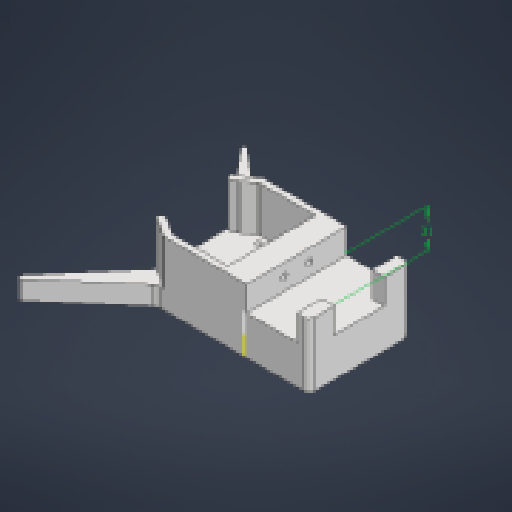
# Autodesk Inventor part: KeChan
Saved by Autodesk Inventor 2027 (Build 310192060, 192F)
## iProperties
Created: 2026-08-23
Part Number: KeChan
Material: Generic
Document SubType Name: Modeling
Designer: trtrn
Density: 1 g/cm^3
Appearance: Default
Author: trtrn
Autodesk Inventor part; units mm, degrees
ref_plane "YZ Plane" through (0, 0, 0) normal (1, 0, 0) x (0, 1, 0)
ref_plane "XZ Plane" through (0, 0, 0) normal (0, 1, 0) x (-1, 0, 0)
ref_plane "XY Plane" through (0, 0, 0) normal (0, 0, 1) x (1, 0, 0)
sketch "Sketch38" plane through (0, 0, 0) normal (0, 1, 0) x (-1, 0, 0)
  line L0 (40, 40) -> (-40, 40)
  line L1 (-40, 40) -> (-40, -40)
  line L2 (-40, -40) -> (40, -40)
  line L3 (40, -40) -> (40, 40)
  line L4 (40, 40) -> (-40, -40) construction
  line L5 (-40, 40) -> (40, -40) construction
  point P0 (0, 0)
  dimension "d203" = 80
  dimension "d204" = 80
  constraints: 12 end point, 2 midpoint, 2 parallel, 1 horizontal, 1 perpendicular
  measures "d203" distance of L2.end L1.end
  measures "d204" distance of L1.end L0.end
extrude "Extrusion36" add sketch "Sketch38" along normal blind 15
sketch "Sketch39" plane through (0, 0, 0) normal (0, -1, 0) x (1, 0, 0)
  line L0 (-35, -35) -> (35, -35)
  line L1 (35, -35) -> (35, 35)
  line L2 (35, 35) -> (-35, 35)
  line L3 (-35, 35) -> (-35, -35)
  line L4 (-35, -35) -> (35, 35) construction
  line L5 (35, -35) -> (-35, 35) construction
  point P0 (0, 0)
  dimension "d207" = 70
  dimension "d208" = 70
  constraints: 12 end point, 2 midpoint, 2 parallel, 1 horizontal, 1 perpendicular
  measures "d207" distance of L2.end L1.end
  measures "d208" distance of L1.end L0.end
extrude "Extrusion37" cut sketch "Sketch39" against normal blind 6
fillet "Fillet5" radius 8 4 edges at (-40, 7.5, -40) (40, 7.5, -40) (40, 7.5, 40) (-40, 7.5, 40)
sketch "Sketch43" plane through (0, 15, 0) normal (0, 1, 0) x (1, 0, 0)
  arc A0 (-32, 40) -> (-40, 32) centre (-32, 32) ccw projected
  arc A1 (-26.7833, 38.0652) -> (-38.0652, 26.7833) centre (-32, 32) ccw
  line L0 (-38.0652, 26.7833) -> (-90.0848, 87.2644)
  line L1 (-87.2644, 90.0848) -> (-26.7833, 38.0652)
  line L2 (0, 0) -> (-32, 32) construction
  arc A2 (-87.2644, 90.0848) -> (-90.0848, 87.2644) centre (-88.5685, 88.5685) ccw
  line L3 (32, 40) -> (-32, 40) projected
  line L4 (-29.0329, 40) -> (-32, 40) construction
  line L5 (-40, 32) -> (-40, -32) projected
  point P0 (-107.4247, 107.4247)
  point P1 (-40, 29.0329)
  dimension "d231" = 2
  dimension "d232" = 80
  constraints: 8 end point, 4 point on circle, 4 point on line, 4 tangent, 2 centre point, 1 coincident, 1 collinear, 1 concentric
  measures "d231" radius of A2
  measures "d232" distance of A2.centre A0.centre
extrude "Extrusion40" add sketch "Sketch43" against normal up to surface (15 mm away) contours A0 L5 L0 A2 L1 L3
pattern_circular "Circular Pattern1" count 2 over 90 about axis through (0, -10, 0) along (0, 1, 0) of "Extrusion40"
fillet "Fillet7" radius 8 4 edges at (-29.0329, 7.5, 40) (-40, 7.5, 29.0329) (-40, 7.5, -29.0329) (-29.0329, 7.5, -40)
sketch "Sketch44" plane through (0, 6, 0) normal (0, -1, 0) x (1, 0, 0)
  circle A0 centre (-17.5, 29) radius 1.65
  circle A1 centre (12.5, 29) radius 1.65
  circle A2 centre (12.5, -29) radius 1.65
  circle A3 centre (-17.5, -29) radius 1.65
  point P0 (0, 0)
  constraints: 4 centre point, 4 coincident, 8 other
hole "Hole3" at (-17.5, 6, -29) at (-17.5, 6, 29) at (12.5, 6, 29) at (12.5, 6, -29) direction (0, 1, 0) diameter 4.3 end through all counterbore diameter 7.52 counterbore depth 4
sketch "Sketch46" plane through (40, 0, 32) normal (1, 0, 0) x (0, 0, -1)
  line L0 (64, 15) -> (64, 0) projected
  line L1 (0, 15) -> (64, 15) projected
  line L2 (0, 0) -> (64, 0) projected
  line L3 (0, 0) -> (0, 15) projected
  line L4 (72, 0) -> (72, 15) projected
  line L5 (72, 0) -> (64, 0) projected
  line L6 (64, 15) -> (72, 15) projected
  line L7 (-8, 15) -> (-8, 0) projected
  line L8 (0, 0) -> (-8, 0) projected
  line L9 (-8, 15) -> (0, 15) projected
  line L10 (-8, 15) -> (72, 15)
  line L11 (72, 15) -> (72, 31)
  line L12 (72, 31) -> (-8, 31)
  line L13 (-8, 31) -> (-8, 15)
  point P0 (32, 0)
  dimension "d254" = 31
  constraints: 8 end point, 2 parallel, 1 collinear, 1 horizontal, 1 perpendicular
  measures "d254" distance between parallel lines of L2 L12
extrude "Extrusion41" add sketch "Sketch46" against normal blind 10 contours L6 L4 L5 L0 | L3 L8 L7 L9
sketch "Sketch47" plane through (0, 15, 0) normal (0, 1, 0) x (1, 0, 0)
  line L0 (22, 8) -> (22, 28)
  line L1 (22, -28) -> (22, -8)
  line L2 (-7.5, -35) -> (-2.5, -35)
  line L3 (-2.5, 35) -> (-7.5, 35)
  line L4 (-7.5, -35) -> (22, -35)
  line L5 (22, -35) -> (22, 35)
  line L6 (22, 35) -> (-7.5, 35)
  line L7 (-7.5, -35) -> (-23, -35)
  line L8 (-7.5, 35) -> (-23, 35)
  line L9 (-26.0657, -40) -> (40, -40) projected
  line L10 (40, 40) -> (-26.0657, 40) projected
  arc A0 (-31.2824, 41.9348) -> (-26.0657, 40) centre (-26.0657, 48) ccw projected
  line L11 (-31.2824, 41.9348) -> (-87.2644, 90.0848) projected
  arc A1 (-26.0657, -40) -> (-31.2824, -41.9348) centre (-26.0657, -48) ccw projected
  line L12 (-87.2644, -90.0848) -> (-31.2824, -41.9348) projected
  line L13 (-90.0848, 87.2644) -> (-41.9348, 31.2824) construction
  line L14 (-32.4052, 28.1827) -> (-36.8295, 26.1921)
  arc A2 (-22.6108, 32.1002) -> (-23, 31.3085) centre (-22, 31.3085) ccw construction
  line L15 (-23, 35) -> (-32.4052, 28.1827)
  line L16 (-38.8811, 30.7518) -> (-34.9244, 32.532)
  line L17 (-34.9244, 32.532) -> (-24.6215, 40)
  line L18 (-24.6215, 40) -> (-7.5, 40)
  line L19 (-7.5, 40) -> (27, 40)
  line L20 (27, 40) -> (27, -40)
  line L21 (27, -40) -> (-7.5, -40)
  line L22 (71.2863, 0) -> (-71.2863, 0) construction
  line L23 (-7.5, -35) -> (-23, -35)
  line L24 (-32.4052, -28.1827) -> (-36.8295, -26.1921)
  line L25 (-23, -35) -> (-32.4052, -28.1827)
  line L26 (-38.8811, -30.7518) -> (-34.9244, -32.532)
  line L27 (-34.9244, -32.532) -> (-24.6215, -40)
  line L28 (-36.8295, 26.1921) -> (-40, 24.7656)
  line L29 (-40, 26.0657) -> (-40, -26.0657) projected
  arc A3 (-40, 26.0657) -> (-41.9348, 31.2824) centre (-48, 26.0657) ccw projected
  line L30 (-38.8811, 30.7518) -> (-40.9388, 29.826)
  line L31 (-36.8295, -26.1921) -> (-40, -24.7656)
  line L32 (-38.8811, -30.7518) -> (-40.9388, -29.826)
  arc A4 (-41.9348, -31.2824) -> (-40, -26.0657) centre (-48, -26.0657) ccw projected
  line L33 (-41.9348, -31.2824) -> (-90.0848, -87.2644) construction
  point P0 (0, 0)
  point P1 (22, -8)
  point P2 (27, -40)
  dimension "d248" = 5
  constraints: 54 end point, 8 symmetric about line, 5 collinear, 5 horizontal, 3 point on circle, 2 parallel, 2 perpendicular, 2 vertical, 2 vertical alignment, 1 centre point, 1 midpoint, 1 point on line, 20 other
  measures "d248" distance between parallel lines of L15 L17
extrude "Extrusion42" add sketch "Sketch47" along normal blind 36 contours L0 L5 L6 L3 L8 L15 L14 L28 L29 A3 L30 L16 L17 L10 L20 L9 L27 L26 L32 A4 L31 L24 L25 L7 L2 L4 L1
fillet "Fillet8" radius 2 10 edges at (-40.9388, 33, -29.826) (-40, 33, -24.7656) (-40, 33, 24.7656) (-40.9388, 33, 29.826) (-24.6215, 33, -40) (-34.9244, 33, -32.532) (-32.4052, 33, -28.1827) (-23, 33, -35) (-23, 33, 35) (-24.6215, 33, 40)
fillet "Fillet9" radius 2 2 edges at (-34.9244, 33, 32.532) (-32.4052, 33, 28.1827)
extrude "Extrusion43" add sketch "Sketch46" against normal up to surface (13 mm away) contours L1 L9 L13 L12 L11 L6
extrude "Extrusion44" add sketch "Sketch46" along normal blind 52
sketch "Sketch48" plane through (27, 51, 40) normal (1, 0, 0) x (0, 0, -1)
  line L0 (0, 0) -> (80, 0) projected
  line L1 (80, -20) -> (80, 0) projected
  line L2 (80, -20) -> (0, -20) projected
  line L3 (0, -20) -> (0, 0) projected
  point P0 (40, -51)
extrude "Extrusion45" add sketch "Sketch48" along normal blind 15
sketch "Sketch49" plane through (22, 15, -35) normal (-1, 0, 0) x (0, 0, 1)
  line L0 (35, -15) -> (35, 64.5533) construction
  line L1 (8.9343, -15) -> (61.0657, -15) projected
  point P0 (25, 26)
  point P1 (45, 26)
  point P2 (35, -15)
  dimension "d261" = 20
  dimension "d262" = 41
  constraints: 2 end point, 1 midpoint, 1 symmetric about line, 1 vertical
  measures "d261" distance of point (25, 26) point (45, 26)
  measures "d262" vertical distance of point (35, -15) point (45, 26)
hole "Hole4" at (22, 41, -10) at (22, 41, 10) direction (1, 0, 0) diameter 5.3 end through all counterbore diameter 9 counterbore depth 5
sketch "Sketch50" plane through (92, 31, 40) normal (0, 1, 0) x (1, 0, 0)
  line L0 (-50, 0) -> (0, 0) projected
  line L1 (-50, 80) -> (0, 80) projected
  line L2 (0, 0) -> (-10, 0)
  line L3 (-10, 0) -> (-10, 80)
  line L4 (-10, 80) -> (0, 80)
  line L5 (0, 80) -> (0, 0)
  point P0 (-92, 40)
  dimension "d270" = 10
  constraints: 8 end point, 2 parallel, 1 horizontal, 1 perpendicular, 1 point on line
  measures "d270" distance of L3.end L4.end
extrude "Extrusion46" add sketch "Sketch50" along normal blind 20
fillet "Fillet11" radius 4 2 edges at (92, 25.5, 40) (92, 25.5, -40)
sketch "Sketch51" plane through (0, 0, 0) normal (0, -1, 0) x (1, 0, 0)
  line L0 (30, -35) -> (-35, -35) projected
  line L1 (-35, 35) -> (30, 35) projected
  line L2 (30, -35) -> (87, -35)
  line L3 (87, -35) -> (87, 35)
  line L4 (87, 35) -> (30, 35)
  line L5 (30, 35) -> (30, -35)
  line L6 (92, 36) -> (92, -36) projected
  line L7 (22, -35) -> (22, 35) projected
  line L8 (-159.4505, 0) -> (159.4505, 0) construction
  line L9 (-25, 15) -> (77, 15)
  line L10 (77, 15) -> (77, -15)
  line L11 (77, -15) -> (-25, -15)
  line L12 (-25, -15) -> (-25, 15)
  line L13 (-35, -35) -> (-35, 35) projected
  line L14 (82, 20) -> (-30, 20)
  line L15 (-30, 20) -> (-30, -20)
  line L16 (-30, -20) -> (82, -20)
  line L17 (82, -20) -> (82, 20)
  point P0 (0, 0)
  point P1 (30, -15)
  point P2 (30, -20)
  point P3 (30, 20)
  point P4 (30, 15)
  dimension "d274" = 5
  dimension "d277" = 30
  dimension "d278" = 10
  dimension "d279" = 10
  dimension "d280" = 5
  constraints: 26 end point, 6 parallel, 3 horizontal, 3 perpendicular, 1 collinear, 1 midpoint, 4 other
  measures "d274" distance between parallel lines of L3 L6
  measures "d277" distance between parallel lines of L11 L9
  measures "d278" distance between parallel lines of L3 L10
  measures "d279" distance between parallel lines of L13 L12
  measures "d280" distance between parallel lines of L9 L14
extrude "Extrusion47" cut sketch "Sketch51" against normal blind 20 contours L5 L16 L17 L14 L4 L3 L2 | L5 L11 L10 L9 L14 L17 L16 | L5 L9 L10 L11
extrude "Extrusion48" add sketch "Sketch51" against normal up to surface (20 mm away) contours L5 L11 L10 L9 L14 L17 L16
extrude "Extrusion49" add sketch "Sketch51" against normal up to surface (6 mm away) contours L16 L7 L11 L5 | L16 L15 L14 L7 L9 L12 L11 | L9 L7 L14 L5
sketch "Sketch52" plane through (92, 0, 32) normal (1, 0, 0) x (0, 0, -1)
  line L0 (32, 53.1826) -> (32, -53.1826) construction
  line L1 (67, 51) -> (-3, 51) projected
  line L2 (12, 51) -> (52, 51)
  line L3 (52, 51) -> (52, 31)
  line L4 (52, 31) -> (12, 31)
  line L5 (12, 31) -> (12, 51)
  line L6 (-8, 31) -> (72, 31) projected
  point P0 (32, 0)
  dimension "d285" = 40
  constraints: 10 end point, 2 parallel, 1 collinear, 1 horizontal, 1 midpoint, 1 perpendicular, 1 point on line, 1 vertical, 1 other
  measures "d285" distance between parallel lines of L5 L3
extrude "Extrusion50" cut sketch "Sketch52" against normal blind 10
sketch "Sketch54" plane through (42, 31, 40) normal (0, 1, 0) x (1, 0, 0)
  line L0 (0, 80) -> (0, 0) projected
  line L1 (40, 80) -> (40, 60) projected
  line L2 (40, 20) -> (40, 0) projected
  line L3 (0, 80) -> (0, 130.5685)
  line L4 (0, 130.5685) -> (40, 130.5685)
  line L5 (40, 130.5685) -> (40, 80)
  line L6 (0, 80) -> (40, 80) projected
  arc A0 (-129.2644, 130.0848) -> (-132.0848, 127.2644) centre (-130.5685, 128.5685) ccw projected
  line L7 (-180.0301, 40) -> (96.0301, 40) construction
  line L8 (0, 0) -> (0, -50.5685)
  line L9 (0, -50.5685) -> (40, -50.5685)
  line L10 (40, -50.5685) -> (40, 0)
  line L11 (0, 0) -> (40, 0) projected
  point P0 (-42, 40)
  constraints: 14 end point, 2 horizontal, 2 symmetric about line, 1 collinear, 1 midpoint, 1 tangent, 1 vertical
extrude "Extrusion51" add sketch "Sketch54" against normal up to surface (31 mm away)
sketch "Sketch55" plane through (82, 31, 90.5685) normal (1, 0, 0) x (0, 0, -1)
  line L0 (0, 0) -> (0, -31) projected
  line L1 (0, -5) -> (50.5685, -31)
  line L2 (0, 0) -> (50.5685, 0) projected
  line L3 (50.5685, 20) -> (50.5685, -31) projected
  line L4 (130.5685, -31) -> (130.5685, 20) projected
  line L5 (130.5685, 0) -> (181.1371, 0) projected
  line L6 (181.1371, 0) -> (181.1371, -31) projected
  line L7 (181.1371, -5) -> (130.5685, -31)
  line L8 (50.5685, -31) -> (0, -31) projected
  line L9 (181.1371, -31) -> (130.5685, -31) projected
  point P0 (90.5685, -31)
  dimension "d290" = 5
  dimension "d291" = 5
  constraints: 4 end point, 2 point on line
  measures "d290" distance from line of L2 L1.start
  measures "d291" distance from line of L5 L7.start
extrude "Extrusion52" cut sketch "Sketch55" against normal up to surface (40 mm away) contours L1 L8 L0 | L7 L6 L9
fillet "Fillet12" radius 4 4 edges at (82, 15.5, 40) (42, 15.5, 40) (82, 15.5, -40) (42, 15.5, -40)
sketch "Sketch56" plane through (82, 31, -90.5685) normal (0, 0, -1) x (-1, 0, 0)
  line L0 (0, -5) -> (40, -5) construction
  line L1 (20, 30.3878) -> (20, -40.3878) construction
  line L2 (107, -31) -> (5, -31) projected
  line L3 (5, -31) -> (35, -31)
  line L4 (35, -31) -> (35, -5)
  line L5 (35, -5) -> (5, -5)
  line L6 (5, -5) -> (5, -31)
  line L7 (0, -28.9434) -> (0, -5) projected
  point P0 (82, -31)
  point P1 (20, -5)
  point P2 (35, -31)
  dimension "d295" = 5
  constraints: 10 end point, 2 midpoint, 2 parallel, 2 point on line, 1 horizontal, 1 perpendicular, 1 vertical, 1 other
  measures "d295" distance between parallel lines of L7 L6
extrude "Extrusion53" cut sketch "Sketch56" against normal up to surface (50.5685 mm away)
mirror "Mirror1" about plane through (0, 0, 0) normal (0, 0, 1) of "Extrusion53"
body "Solid2"
